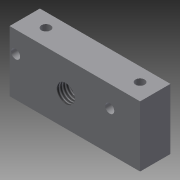
# Autodesk Inventor part: heAluBase
Saved by Autodesk Inventor 2013 (Build 170138000, 138)
## iProperties
Created: 2015-01-15
Part Number: heAluBase
Material: Generic
Document SubType Name: Modeling
Designer: dzban
Density: 1 g/cm^3
Author: dzban
Autodesk Inventor part; units mm, degrees
ref_plane "YZ Plane" through (0, 0, 0) normal (1, 0, 0) x (0, 1, 0)
ref_plane "XZ Plane" through (0, 0, 0) normal (0, 1, 0) x (-1, 0, 0)
ref_plane "XY Plane" through (0, 0, 0) normal (0, 0, 1) x (1, 0, 0)
sketch "Sketch1" plane through (0, 0, 0) normal (0, 0, 1) x (1, 0, 0)
  line L0 (0, 0) -> (43, 0)
  line L1 (43, 0) -> (43, 10)
  line L2 (43, 10) -> (0, 10)
  line L3 (0, 10) -> (0, 0)
  circle A0 centre (6.5, 5.5) radius 1.5
  circle A1 centre (37.5, 5.5) radius 1.5
  dimension "d0" = 43
  dimension "d1" = 10
  dimension "d2" = 3
  dimension "d3" = 3
  dimension "d4" = 6.5
  dimension "d5" = 31
  dimension "d6" = 4.5
  constraints: 8 end point, 2 centre point, 1 horizontal alignment
  measures "d0" distance of L0.start L0.end
  measures "d1" distance of L2.end L0.start
  measures "d2" diameter of A0
  measures "d3" diameter of A1
  measures "d4" distance from line of A0.centre L3
  measures "d5" distance of A1.centre A0.centre
  measures "d6" distance from line of L2 A0.centre
extrude "Extrusion1" add sketch "Sketch1" along normal blind 20
sketch "Sketch2" plane through (0, 10, 0) normal (0, 1, 0) x (1, 0, 0)
  line L0 (0, 0) -> (0, -20) projected
  line L1 (43, -20) -> (0, -20) projected
  circle A0 centre (2, -13) radius 1.5
  circle A1 centre (33, -13) radius 1.5
  dimension "d9" = 7
  dimension "d10" = 2
  dimension "d11" = 3
  dimension "d12" = 3
  dimension "d13" = 31
  constraints: 2 centre point, 1 horizontal alignment
  measures "d9" distance from line of A0.centre L1
  measures "d10" distance from line of A0.centre L0
  measures "d11" diameter of A0
  measures "d12" diameter of A1
  measures "d13" distance of A1.centre A0.centre
extrude "Extrusion2" cut sketch "Sketch2" against normal blind 20
sketch "Sketch3" plane through (0, 10, 0) normal (0, 1, 0) x (1, 0, 0)
  line L0 (0, 0) -> (0, -20) projected
  line L1 (43, -20) -> (0, -20) projected
  circle A0 centre (18.5, -10) radius 3
  dimension "d16" = 6
  dimension "d18" = 10
  dimension "d19" = 18.5
  constraints: 1 centre point
  measures "d16" diameter of A0
  measures "d18" distance from line of A0.centre L1
  measures "d19" distance from line of L0 A0.centre
hole "Hole1" at (18.5, 10, 10) direction (0, -1, 0) diameter 6 depth 0.0001 tip angle 118
sketch "Sketch4" plane through (0, 0, 0) normal (0, -1, 0) x (1, 0, 0)
  line L0 (0, 20) -> (43, 20) projected
  line L1 (0, 0) -> (0, 20) projected
  circle A0 centre (18.5, 10) radius 2.2122
  dimension "d27" = 10
  dimension "d28" = 18.5
  constraints: 1 centre point
  measures "d27" distance from line of L0 A0.centre
  measures "d28" distance from line of A0.centre L1
hole "Hole2" at (18.5, 0, 10) direction (0, 1, 0) diameter 6 depth 8 tip angle 135
thread "Thread1" size "M6x1" class "6H" standard "ANSI Metric M Profile" full length
body "Solid1"
